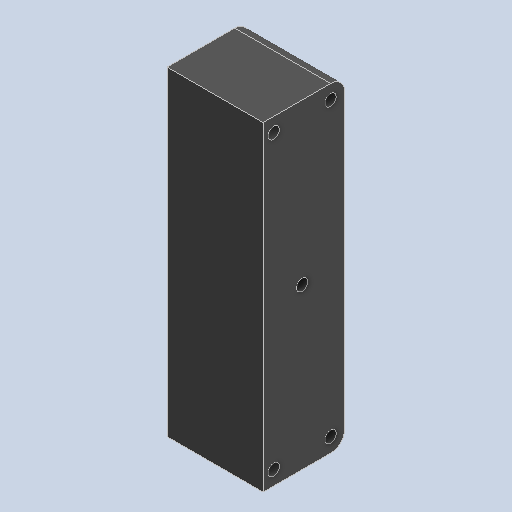
# Autodesk Inventor part: chest_cover_stopper
Saved by Autodesk Inventor 2024.1 (Build 281209000, 209)
## iProperties
Created: 2024-02-15
Part Number: chest_cover_stopper
Material: 一般
Document SubType Name: Modeling
Designer: hibik
Density: 1 g/cm^3
Appearance: 既定
Author: hibik
Autodesk Inventor part; units mm, degrees
ref_plane "YZ Plane" through (0, 0, 0) normal (1, 0, 0) x (0, 1, 0)
ref_plane "XZ Plane" through (0, 0, 0) normal (0, 1, 0) x (-1, 0, 0)
ref_plane "XY Plane" through (0, 0, 0) normal (0, 0, 1) x (1, 0, 0)
sketch "スケッチ1" plane through (0, 0, 0) normal (1, 0, 0) x (0, 1, 0)
  line L0 (45, 0) -> (0, 0)
  line L1 (0, 0) -> (0, -11.5)
  line L2 (0, -11.5) -> (45, -11.5)
  line L3 (45, -11.5) -> (45, 0)
  dimension "d0" = 45
  dimension "d1" = 11.5
  constraints: 8 end point, 2 parallel, 1 coincident, 1 horizontal, 1 perpendicular
  measures "d0" distance of L0.start L0.end
  measures "d1" distance of L2.end L0.start
extrude "押し出し1" add sketch "スケッチ1" along normal blind 13.5
sketch "スケッチ2" plane through (13.5, 0, 0) normal (1, 0, 0) x (0, 0, -1)
  circle A0 centre (1.5, 43) radius 0.8 projected
  circle A1 centre (9.4807, 43) radius 0.8 projected
  circle A2 centre (9.5, 2) radius 0.8 projected
  circle A3 centre (1.5, 2) radius 0.8 projected
  circle A4 centre (5.5, 22.5) radius 0.8 projected
  point P0 (0, 0)
extrude "押し出し2" cut sketch "スケッチ2" against normal through all
fillet "フィレット1" radius 2 2 edges at (6.75, 45, -11.5) (6.75, 0, -11.5)
